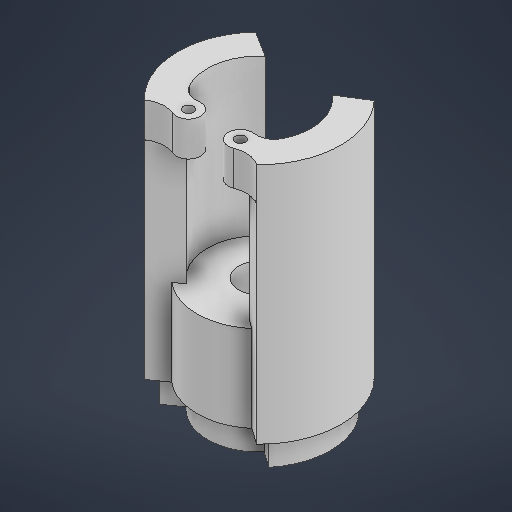
# Autodesk Inventor part: 가변저항 고정
Saved by Autodesk Inventor 2026.2 (Build 302298000, 298)
## iProperties
Created: 2025-11-20
Part Number: 가변저항 고정
Material: 일반
Document SubType Name: Modeling
Designer: PC
Density: 1 g/cm^3
Appearance: 기본값
Author: PC
Autodesk Inventor part; units mm, degrees
ref_plane "YZ Plane" through (0, 0, 0) normal (1, 0, 0) x (0, 1, 0)
ref_plane "XZ Plane" through (0, 0, 0) normal (0, 1, 0) x (-1, 0, 0)
ref_plane "XY Plane" through (0, 0, 0) normal (0, 0, 1) x (1, 0, 0)
sketch "스케치1" plane through (0, 0, 0) normal (0, 1, 0) x (-1, 0, 0)
  circle A0 centre (0, 0) radius 6
  circle A1 centre (0, 0) radius 20.5
  line L0 (4.1418, -4.3412) -> (16.542, -12.1084)
  line L1 (0, -28.7) -> (0, 28.7) projected
  line L2 (-4.1418, -4.3412) -> (-16.542, -12.1084)
  line L3 (15.8025, 13.0588) -> (3.8109, 4.6343)
  circle A2 centre (0, 0) radius 15
  line L4 (-15.8025, 13.0588) -> (-3.8109, 4.6343)
  point P0 (11.2832, 9.8838)
  point P1 (-11.2832, 9.8838)
  point P2 (-15.8025, 13.0588)
  point P3 (-16.542, -12.1084)
  dimension "d0" = 12
  dimension "d1" = 41
  dimension "d2" = 30
  constraints: 8 end point, 4 point on circle, 4 symmetric about line, 3 centre point, 3 coincident
  measures "d0" diameter of A0
  measures "d1" diameter of A1
  measures "d2" diameter of A2
extrude "돌출1" add sketch "스케치1" along normal blind 8 contours A0 L3 A2 L0 | A0 L1 A2 L3 | A0 L4 A2 L1 | L3 A1 L0 A2 | A0 L2 A2 L4 | A2 L2 A1 L4
sketch "스케치3" plane through (0, 8, 0) normal (0, 1, 0) x (1, 0, 0)
  circle A0 centre (0, 0) radius 23.5
  arc A1 (-4.1418, 4.3412) -> (4.1418, 4.3412) centre (0, 0) ccw projected
  circle A2 centre (0, 0) radius 6
  line L0 (-15.8025, -13.0588) -> (-11.2832, -9.8838) projected
  arc A3 (-11.2832, -9.8838) -> (11.2832, -9.8838) centre (0, 0) ccw projected
  arc A4 (-16.542, 12.1084) -> (-15.8025, -13.0588) centre (0, 0) ccw projected
  line L1 (11.2832, -9.8838) -> (15.8025, -13.0588) projected
  arc A5 (15.8025, -13.0588) -> (16.542, 12.1084) centre (0, 0) ccw projected
  arc A6 (16.2118, -17.0126) -> (18.9628, 13.8803) centre (0, 0) ccw
  line L2 (16.2118, -17.0126) -> (11.5942, -13.7686)
  arc A7 (-11.5942, -13.7686) -> (11.5942, -13.7686) centre (0, 0) ccw
  line L3 (-11.5942, -13.7686) -> (-16.2118, -17.0126)
  arc A8 (-18.9628, 13.8803) -> (-16.2118, -17.0126) centre (0, 0) ccw
  line L4 (-4.1418, 4.3412) -> (-16.542, 12.1084) projected
  line L5 (16.542, 12.1084) -> (4.1418, 4.3412) projected
  line L6 (-17.1719, 16.0429) -> (-1.0036, 5.9155)
  line L7 (0, 0) -> (0, 6)
  line L8 (17.1719, 16.0429) -> (1.0036, 5.9155)
  circle A9 centre (0, 0) radius 9
  point P0 (4.1418, 4.3412)
  point P1 (-4.2366, 7.9405)
  point P2 (16.2118, -17.0126)
  point P3 (4.2366, 7.9405)
  dimension "d8" = 47
  dimension "d12" = 3
  dimension "d13" = 3
  constraints: 10 end point, 10 point on circle, 6 centre point, 3 coincident, 2 symmetric about line, 1 concentric, 1 parallel, 1 vertical, 4 other
  measures "d8" diameter of A0
  measures "d12" distance between parallel lines of L6 L4
  measures "d13" radial gap between concentric circles of A9 A2
extrude "돌출3" add sketch "스케치3" along normal blind 25 contours A0 L2 A7 L3 L6 A9 L4 A4 L0 A3 L1 A5 L5 L8 | A9 L5 A2 L8 | L8 A2 L6 A9 | L6 A2 L4 A9 | A9 L4 A1 L5 | L5 A5 L1 A3 L0 A4 L4 A9
sketch "스케치4" plane through (0, 33, 0) normal (0, 1, 0) x (1, 0, 0)
  circle A0 centre (0, 0) radius 15
  line L0 (-16.2118, -17.0126) -> (-9.037, -11.9721)
  line L1 (-16.2118, -17.0126) -> (-11.5942, -13.7686) projected
  arc A1 (16.2118, -17.0126) -> (17.1719, 16.0429) centre (0, 0) ccw projected
  line L2 (16.2118, -17.0126) -> (9.037, -11.9721)
  line L3 (11.5942, -13.7686) -> (16.2118, -17.0126) projected
  line L4 (-4.2366, 7.9405) -> (-17.1719, 16.0429) projected
  arc A2 (-17.1719, 16.0429) -> (-16.2118, -17.0126) centre (0, 0) ccw projected
  line L5 (17.1719, 16.0429) -> (4.2366, 7.9405) projected
  point P0 (9.7534, 11.3961)
  point P1 (-9.7534, 11.3961)
  dimension "d14" = 30
  constraints: 4 end point, 2 collinear, 2 point on circle, 1 centre point, 1 coincident
  measures "d14" diameter of A0
extrude "돌출4" add sketch "스케치4" along normal blind 45 contours L0 A2 L4 A0 | A0 L5 A1 L2
sketch "스케치5" plane through (0, 78, 0) normal (0, 1, 0) x (1, 0, 0)
  circle A0 centre (-7.5, -13) radius 1.5
  circle A1 centre (7.5, -13) radius 1.5
  line L0 (-7.5, -13) -> (7.5, -13)
  line L1 (0, 23.9029) -> (0, -31.1174) projected
  line L2 (-16.2118, -17.0126) -> (-9.037, -11.9721) projected
  arc A2 (-9.7534, 11.3961) -> (-9.037, -11.9721) centre (0, 0) ccw projected
  line L3 (-9.7534, 11.3961) -> (-17.1719, 16.0429) projected
  arc A3 (-17.1719, 16.0429) -> (-16.2118, -17.0126) centre (0, 0) ccw projected
  circle A4 centre (-7.5, -13) radius 3.5
  arc A5 (-13.3097, -6.9175) -> (-8.0654, -9.546) centre (-8.8731, -4.6116) ccw
  arc A6 (-9.7534, 11.3961) -> (-9.037, -11.9721) centre (0, 0) ccw projected
  arc A7 (-8.8597, -16.2251) -> (-16.2118, -17.0126) centre (-11.8247, -23.2573) ccw
  line L4 (-16.2118, -17.0126) -> (-9.037, -11.9721) projected
  circle A8 centre (7.5, -13) radius 3.5
  arc A9 (8.0654, -9.546) -> (13.3097, -6.9175) centre (8.8731, -4.6116) ccw
  arc A10 (16.2118, -17.0126) -> (8.8597, -16.2251) centre (11.8247, -23.2573) ccw
  arc A11 (9.037, -11.9721) -> (9.7534, 11.3961) centre (0, 0) ccw projected
  line L5 (9.037, -11.9721) -> (16.2118, -17.0126) projected
  point P0 (0, -13)
  dimension "d17" = 3
  dimension "d18" = 3
  dimension "d19" = 15
  dimension "d20" = 13
  dimension "d21" = 2
  dimension "d22" = 5
  constraints: 13 point on circle, 8 centre point, 6 symmetric about line, 4 tangent, 2 end point, 1 horizontal, 1 midpoint, 1 point on line, 3 other
  measures "d17" diameter of A0
  measures "d18" diameter of A1
  measures "d19" distance of L0.end L0.start
  measures "d20" distance from line of point (0, 0) L0
  measures "d21" radial gap between concentric circles of A0 A4
  measures "d22" radius of A5
extrude "돌출5" add sketch "스케치5" against normal blind 10 contours A4 L2 A2 | A8 A11 L5 | A4 A2 A5 | A7 L2 A4 | A9 A11 A8 | A8 L5 A10 picked at (-9.0463, -11.1348) picked at (9.0463, -11.1348)
